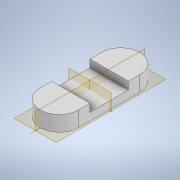
# Autodesk Inventor part: Tile_Connector
Saved by Autodesk Inventor 2022.4 (Build 264492010, 492A)
## iProperties
Created: 2025-02-20
Part Number: Tile_Connector
Material: Generic
Document SubType Name: Modeling
Designer: jan-m
Density: 1 g/cm^3
Appearance: Default
Author: jan-m
Autodesk Inventor part; units mm, degrees
sketch "Sketch1" plane through (0, 0, 0) normal (0, 1, 0) x (-1, 0, 0)
  line L0 (5, 0) -> (-5, 0)
  line L1 (-5, 0) -> (-5, 8)
  line L2 (-5, 8) -> (5, 8)
  line L3 (5, 8) -> (5, 0)
  line L4 (0, -18.2) -> (0, 18.2) projected
  line L5 (7, 0) -> (-7, 0) projected
  line L6 (5, 5) -> (-5, 5)
  arc A0 (5, 8) -> (-5, 8) centre (0, 8) ccw
  line L7 (-5, 0) -> (-5, -8)
  line L8 (-5, -8) -> (5, -8)
  line L9 (5, -8) -> (5, 0)
  line L10 (5, -5) -> (-5, -5)
  arc A1 (-5, -8) -> (5, -8) centre (0, -8) ccw
  point P0 (0, 0)
  point P1 (0, 8)
  dimension "d0" = 10
  dimension "d1" = 8
  dimension "d2" = 3
  constraints: 18 end point, 5 point on line, 5 symmetric about line, 4 point on circle, 2 centre point, 2 parallel, 2 perpendicular, 2 tangent, 1 collinear, 1 horizontal, 1 midpoint, 1 other
  measures "d0" distance of L0.start L0.end
  measures "d1" distance of L2.end L0.start
  measures "d2" distance between parallel lines of L2 L6
extrude "Extrusion1" add sketch "Sketch1" along normal blind 2 contours L9 L10 L4 L0 | L0 L4 L6 L3 | L4 L10 L7 L0 | L0 L1 L6 L4
extrude "Extrusion2" add sketch "Sketch1" along normal blind 4 contours L6 L4 L2 L3 | L9 L8 L4 L10 | L4 L8 L7 L10 | L6 L1 L2 L4 | L2 L4 A0 | A1 L4 L8 | L4 A1 L8 | L2 A0 L4
body "Solid1"
